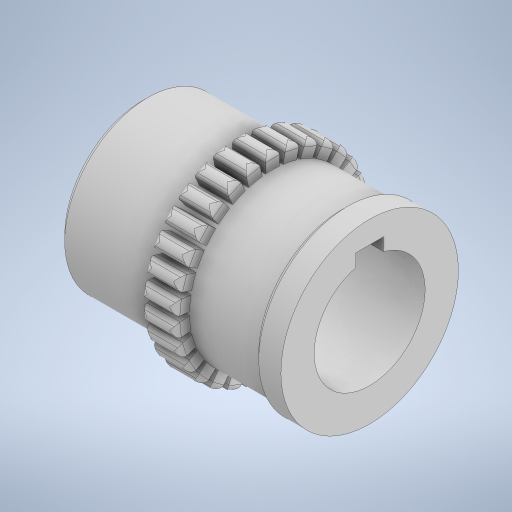
# Autodesk Inventor part: koło zębate
Saved by Autodesk Inventor 2024 (Build 280153000, 153)
## iProperties
Created: 2023-11-21
Part Number: koło zębate
Material: Ogólny
Document SubType Name: Modeling
Designer: Wojciech
Density: 1 g/cm^3
Appearance: Domyślna
Author: Wojciech
Autodesk Inventor part; units mm, degrees
ref_plane "XZ Plane" through (0, 0, 0) normal (0, 1, 0) x (-1, 0, 0)
ref_plane "XY Plane" through (0, 0, 0) normal (0, 0, 1) x (1, 0, 0)
sketch "Szkic1" plane through (0, 0, 0) normal (1, 0, 0) x (0, 1, 0)
  circle A0 centre (0, 0) radius 20
  line L0 (24, 5) -> (16, 5)
  line L1 (16, 5) -> (16, -5)
  line L2 (16, -5) -> (24, -5)
  line L3 (24, -5) -> (24, 5)
  line L4 (24, 5) -> (16, -5) construction
  line L5 (16, 5) -> (24, -5) construction
  circle A1 centre (0, 0) radius 30
  point P0 (20, 0)
  point P1 (19.3649, -5)
  point P2 (19.3649, 5)
  dimension "d0" = 40
  dimension "d1" = 8
  dimension "d2" = 10
  dimension "d3" = 60
  constraints: 12 end point, 2 coincident, 2 midpoint, 2 parallel, 1 centre point, 1 horizontal, 1 horizontal alignment, 1 perpendicular, 3 other
  measures "d1" distance of L2.end L1.end
  measures "d2" distance of L1.end L0.end
  measures "d3" diameter of A1
extrude "Wyciągnięcie proste1" add sketch "Szkic1" against normal blind 82
ref_plane "Płaszczyzna konstrukcyjna1" through (-41, 0, 0) normal (1, 0, 0) x (0, 1, 0)
sketch "Szkic2" plane through (-41, 0, 0) normal (1, 0, 0) x (0, 1, 0)
  circle A0 centre (0, 0) radius 30 projected
  line L0 (30, 0) -> (35.4, 0)
  line L1 (35.4, 0) -> (35.4, -2.5)
  line L2 (24, -5) -> (24, 5) projected
  line L3 (35.4, 0) -> (35.4, 2.5)
  line L4 (35.4, 2.5) -> (29.8957, 2.5)
  line L5 (35.4, -2.5) -> (29.8957, -2.5)
  line L6 (34.0432, 2.5) -> (34.0432, -2.5) construction
  line L7 (34.0432, 2.5) -> (39.0432, 2.5) construction
  dimension "d7" = 5.4
  dimension "d8" = 2.5
  dimension "d9" = 5.5043
  dimension "d10" = 90
  constraints: 14 end point, 3 horizontal, 2 point on circle, 2 point on line, 2 symmetric about line, 1 parallel, 1 perpendicular
  measures "d7" distance of L0.start L0.end
  measures "d8" distance of L0.end L1.end
  measures "d9" distance of L3.end L4.end
  measures "d10" angle of L6 L7
extrude "Wyciągnięcie proste2" add sketch "Szkic2" along normal mid plane 12 contours L0 L1 L5 A0 | A0 L4 L3 L0
sketch "Szkic4" plane through (-47, 0, 0) normal (-1, 0, 0) x (0, 0, 1)
  line L0 (2.5, 29.8957) -> (2.5, 35.4) projected
  line L1 (-2.5, 35.4) -> (-2.5, 29.8957) projected
  arc A0 (1.6736, 34.8574) -> (-1.6736, 34.8574) centre (0, 32.5479) ccw
  line L2 (-2.5, 33.9207) -> (2.5, 33.9207) construction
  line L3 (-2.5, 33.9207) -> (2.5, 33.9207) construction
  line L4 (-2.5, 35.4) -> (0, 35.4)
  line L5 (2.5, 35.4) -> (-2.5, 35.4) projected
  line L6 (0, 35.4) -> (2.5, 35.4)
  line L7 (-2.5, 33.2379) -> (-2.5, 29.8957)
  line L8 (2.5, 33.2379) -> (2.5, 29.8957)
  arc A1 (-1.6736, 34.8574) -> (-2.5, 33.2379) centre (-0.5, 33.2379) ccw
  arc A2 (2.5, 33.2379) -> (1.6736, 34.8574) centre (0.5, 33.2379) ccw
  point P0 (0, 0)
  dimension "d22" = 0
  dimension "d23" = 2
  constraints: 12 end point, 8 point on circle, 5 tangent, 4 point on line, 3 centre point, 2 collinear, 1 equal radius, 1 horizontal, 1 midpoint, 1 perpendicular
  measures "d22" distance between parallel lines of L2 L3
  measures "d23" radius of A1
extrude "Wyciągnięcie proste4" cut sketch "Szkic4" against normal blind 24.25
sketch "Szkic5" plane through (0, 0, 0) normal (0, 0, 1) x (1, 0, 0)
  line L0 (-35, 35.4) -> (-47, 35.4) projected
  line L1 (-47, 29.8957) -> (-47, 33.2379) projected
  line L2 (-35, 33.2379) -> (-35, 29.8957) projected
  line L3 (-47, 34.8574) -> (-47, 33.2379) projected
  line L4 (-47, 35.4) -> (-47, 34.8574) projected
  line L5 (-35, 34.8574) -> (-35, 35.4) projected
  line L6 (-35, 33.2379) -> (-35, 34.8574) projected
  line L7 (0, 30) -> (-82, 30) projected
  line L8 (-47, 30) -> (-47, 33.4)
  line L9 (-37, 35.4) -> (-45, 35.4)
  line L10 (-35, 33.4) -> (-35, 30)
  arc A0 (-35, 33.4) -> (-37, 35.4) centre (-37, 33.4) ccw
  arc A1 (-45, 35.4) -> (-47, 33.4) centre (-45, 33.4) ccw
  point P0 (0, 0)
  dimension "d26" = 2
  constraints: 8 point on line, 6 end point, 4 point on circle, 4 tangent, 2 centre point, 2 collinear, 1 equal radius
  measures "d26" radius of A0
extrude "Wyciągnięcie proste5" cut sketch "Szkic5" along normal mid plane 12.25 contours L5 L6 A0 L0 | A1 L3 L4 L0
pattern_circular "Szyk kołowy2" count 30 over 360 about axis through (-10, 0, 0) along (1, 0, 0) of "Wyciągnięcie proste2", "Wyciągnięcie proste4", "Wyciągnięcie proste5"
sketch "Szkic6" plane through (0, 0, 0) normal (0, 0, 1) x (1, 0, 0)
  line L0 (0, -30) -> (0, 30) projected
  line L1 (0, 30) -> (-82, 30) projected
  line L2 (0, 30) -> (0, 32)
  line L3 (0, 32) -> (-8, 32)
  line L4 (-8, 32) -> (-10, 32)
  line L5 (-10, 32) -> (-10, 30)
  line L6 (-8, 32) -> (-10, 30)
  line L7 (-98.4, 0) -> (16.4, 0) projected
  point P0 (0, 0)
  dimension "d32" = 2
  dimension "d33" = 8
  dimension "d34" = 2
  constraints: 10 end point, 2 perpendicular, 2 point on line, 1 vertical
  measures "d32" distance of L1.start L2.end
  measures "d33" distance of L2.end L3.end
  measures "d34" distance of L3.end L4.end
revolve "Obrót1" add sketch "Szkic6" angle 360 about axis through (-10, 0, 0) along (1, 0, 0) contours L1 L6 L3 L2
chamfer "Faza1" distance 2 angle 45 1 edges at (-82, -30, 0) measured on face at (-82, -29.5, 0)
chamfer "Faza2" distance 1 angle 45 1 edges at (-82, -20, 0) measured on face at (-82, -20.5, 0)
